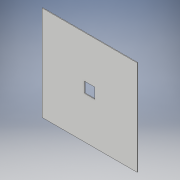
# Autodesk Inventor part: Wall
Saved by Autodesk Inventor 2018 (Build 220112000, 112)
## iProperties
Created: 2019-11-15
Part Number: Wall
Material: Generic
Document SubType Name: Modeling
Designer: Jacob
Density: 1 g/cm^3
Appearance: Default
Author: Jacob
Autodesk Inventor part; units mm, degrees
ref_plane "YZ Plane" through (0, 0, 0) normal (1, 0, 0) x (0, 1, 0)
ref_plane "XZ Plane" through (0, 0, 0) normal (0, 1, 0) x (-1, 0, 0)
ref_plane "XY Plane" through (0, 0, 0) normal (0, 0, 1) x (1, 0, 0)
sketch "Sketch1" plane through (0, 0, 0) normal (0, 0, 1) x (1, 0, 0)
  line L0 (-457.2, 457.2) -> (457.2, 457.2)
  line L1 (457.2, 457.2) -> (457.2, -457.2)
  line L2 (457.2, -457.2) -> (-457.2, -457.2)
  line L3 (-457.2, -457.2) -> (-457.2, 457.2)
  line L4 (-457.2, 457.2) -> (457.2, -457.2) construction
  line L5 (457.2, 457.2) -> (-457.2, -457.2) construction
  line L6 (-50.8, 50.8) -> (50.8, 50.8)
  line L7 (50.8, 50.8) -> (50.8, -50.8)
  line L8 (50.8, -50.8) -> (-50.8, -50.8)
  line L9 (-50.8, -50.8) -> (-50.8, 50.8)
  line L10 (-50.8, 50.8) -> (50.8, -50.8) construction
  line L11 (50.8, 50.8) -> (-50.8, -50.8) construction
  point P0 (0, 0)
  dimension "d0" = 914.4
  dimension "d1" = 914.4
  dimension "d2" = 101.6
  dimension "d3" = 101.6
  constraints: 24 end point, 4 midpoint, 4 parallel, 2 horizontal, 2 perpendicular
  measures "d0" distance of L0.start L0.end
  measures "d1" distance of L0.end L1.end
  measures "d2" distance of L6.end L7.end
  measures "d3" distance of L6.start L6.end
extrude "Extrusion1" add sketch "Sketch1" along normal blind 6.35
body "Solid1"
